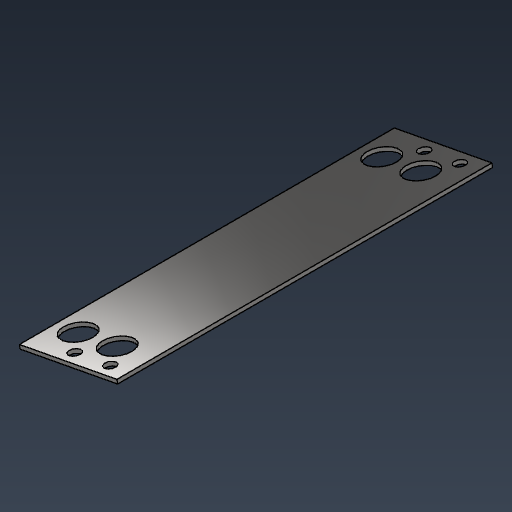
# Autodesk Inventor part: SteelFront
Saved by Autodesk Inventor 2026.2 (Build 302298010, 298A)
## iProperties
Created: 2026-04-07
Part Number: SteelFront
Material: Steel, Alloy
Document SubType Name: Modeling
Designer: szymo
Density: 7.73 g/cm^3
Appearance: Semi-Polished(2)
Mass: 18.6952 g
Surface Area: 52.2825 cm^2
Volume: 2.41853 cm^3
Author: szymo
Autodesk Inventor part; units mm, degrees
ref_plane "YZ Plane" through (0, 0, 0) normal (1, 0, 0) x (0, 1, 0)
ref_plane "XZ Plane" through (0, 0, 0) normal (0, 1, 0) x (-1, 0, 0)
ref_plane "XY Plane" through (0, 0, 0) normal (0, 0, 1) x (1, 0, 0)
sketch "Sketch1" plane through (0, 0, 0) normal (0, 0, 1) x (1, 0, 0)
  line L0 (0, -97) -> (0, -84.632) construction
  line L1 (3, -84.632) -> (3, -92) construction
  line L2 (3, -92) -> (5, -92) construction
  line L3 (5, -92) -> (0, -97) construction
  circle A0 centre (14.5, -55.2958) radius 14.5 construction
  line L4 (3.3867, -91.8) -> (29.4, -86.8578)
  line L5 (29.4, -86.8578) -> (29.2133, -85.8753)
  line L6 (29.2133, -85.8753) -> (3.2, -90.8176)
  line L7 (3.2, -90.8176) -> (3.3867, -91.8)
  line L8 (29.4, -86.8578) -> (29.4, -70.3377) construction
  line L9 (27, -86.2958) -> (6.5, -86.2958) projected
  line L10 (6.5, -86.2958) -> (6.5, -69.7958) projected
  line L11 (27, -69.7958) -> (6.5, -69.7958) projected
  line L12 (27, -86.2958) -> (27, -69.7958) projected
  line L13 (3, -84.632) -> (0, -84.632) projected
  dimension "d0" = 1
  dimension "d1" = 0.2
  dimension "d2" = 0.2
  dimension "d3" = 0.4
  dimension "d4" = 0
  constraints: 10 end point, 2 parallel, 1 perpendicular, 1 vertical
  measures "d0" distance between parallel lines of L6 L4
  measures "d1" distance from line of L1 L6.end
  measures "d2" distance from line of L2 L4.start
  measures "d3" distance edge to line of A0 L8
  measures "d4" distance from line of L6 L9.start
extrude "Extrusion1" add sketch "Sketch1" along normal mid plane 100 contours L7 L6 L5 L4
sketch "Sketch2" plane through (29.4, -86.8578, -50) normal (0.18665, -0.9824265, 0) x (0.9824265, 0.18665, 0)
  line L0 (-23.6286, 15.5) -> (-23.6286, 84.5) projected
  line L1 (-26.6823, 0) -> (-26.6823, 100) projected
  circle A0 centre (-5.2529, 96.6288) radius 1.5
  circle A1 centre (-14.9133, 96.6288) radius 1.5
  circle A2 centre (-14.9133, 3.3712) radius 1.5
  circle A3 centre (-5.2529, 3.3712) radius 1.5
  circle A4 centre (-9.6065, 90.5) radius 4
  circle A5 centre (-20.2202, 90.5) radius 4
  circle A6 centre (-9.6065, 9.5) radius 4
  circle A7 centre (-20.2202, 9.5) radius 4
  circle A8 centre (-14.9133, 96.6288) radius 2.25 projected
  circle A9 centre (-5.2529, 96.6288) radius 2.25 projected
  ellipse E0 centre (-20.2202, 90.5) end of major axis (-15.6671, 90.5) minor radius 4.5 (-16.2752, 92.7467) -> (-16.2752, 88.2533) ccw projected
  line L2 (-16.2752, 92.7467) -> (-13.5515, 92.7467) projected
  ellipse E1 centre (-9.6065, 90.5) end of major axis (-5.0534, 90.5) minor radius 4.5 (-13.5515, 88.2533) -> (-13.5515, 92.7467) ccw projected
  line L3 (-13.5515, 88.2533) -> (-16.2752, 88.2533) projected
  circle A10 centre (-14.9133, 3.3712) radius 2.25 projected
  circle A11 centre (-5.2529, 3.3712) radius 2.25 projected
  ellipse E2 centre (-20.2202, 9.5) end of major axis (-15.6671, 9.5) minor radius 4.5 (-16.2752, 11.7467) -> (-16.2752, 7.2533) ccw projected
  line L4 (-16.2752, 11.7467) -> (-13.5515, 11.7467) projected
  ellipse E3 centre (-9.6065, 9.5) end of major axis (-5.0534, 9.5) minor radius 4.5 (-13.5515, 7.2533) -> (-13.5515, 11.7467) ccw projected
  line L5 (-13.5515, 7.2533) -> (-16.2752, 7.2533) projected
  line L6 (-2.2529, 84.5) -> (-23.6286, 84.5) projected
  line L7 (-2.2529, 84.5) -> (-2.2529, 100) projected
  line L8 (-2.2529, 100) -> (-26.6823, 100) projected
  line L9 (-2.2529, 0) -> (-26.6823, 0) projected
  line L10 (-2.2529, 15.5) -> (-2.2529, 0) projected
  line L11 (-2.2529, 15.5) -> (-23.6286, 15.5) projected
  point P0 (-12.6713, 50)
  dimension "d7" = 3
  dimension "d8" = 3
  dimension "d9" = 3
  dimension "d10" = 3
  dimension "d13" = 8
  dimension "d14" = 8
  dimension "d15" = 8
  dimension "d16" = 8
  constraints: 8 centre point, 4 other
  measures "d7" diameter of A0
  measures "d8" diameter of A1
  measures "d9" diameter of A2
  measures "d10" diameter of A3
  measures "d13" diameter of A4
  measures "d14" diameter of A5
  measures "d15" diameter of A7
  measures "d16" diameter of A6
extrude "Extrusion2" cut sketch "Sketch2" against normal through all contours A0 | A1 | A2 | A3 | A4 | A5 | A6 | A7
equation "\"d14\" = d13"
equation "\"d15\" = d13"
equation "\"d16\" = d13"
body "Solid1"
